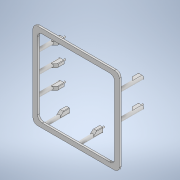
# Autodesk Inventor part: Jig
Saved by Autodesk Inventor 2022.3 (Build 263350030, 350C)
## iProperties
Created: 2023-05-04
Part Number: Jig
Material: Generic
Document SubType Name: Modeling
Designer: Ben
Density: 1 g/cm^3
Appearance: Default
Author: Ben
Autodesk Inventor part; units mm, degrees
(part 1 of 2)
ref_plane "Work Plane1" through (0, 0, 25) normal (0, 0, 1) x (1, 0, 0)
sketch "Sketch1" plane through (0, 0, 25) normal (0, 0, 1) x (1, 0, 0)
  line L0 (46.5, -46.5) -> (-46.5, -46.5)
  line L1 (-46.5, -46.5) -> (-46.5, 46.5)
  line L2 (-46.5, 46.5) -> (46.5, 46.5)
  line L3 (46.5, 46.5) -> (46.5, -46.5)
  line L4 (46.5, -46.5) -> (-46.5, 46.5) construction
  line L5 (-46.5, -46.5) -> (46.5, 46.5) construction
  line L6 (-41.5, 41.5) -> (41.5, 41.5)
  line L7 (41.5, 41.5) -> (41.5, -41.5)
  line L8 (41.5, -41.5) -> (-41.5, -41.5)
  line L9 (-41.5, -41.5) -> (-41.5, 41.5)
  line L10 (-41.5, 41.5) -> (41.5, -41.5) construction
  line L11 (41.5, 41.5) -> (-41.5, -41.5) construction
  point P0 (0, 0)
  dimension "d0" = 93
  dimension "d1" = 93
  dimension "d2" = 83
  dimension "d3" = 83
  constraints: 24 end point, 4 midpoint, 4 parallel, 2 horizontal, 2 perpendicular
  measures "d0" distance of L1.end L2.end
  measures "d1" distance of L0.end L1.end
  measures "d2" distance of L7.end L8.end
  measures "d3" distance of L6.end L7.end
extrude "Extrusion1" add sketch "Sketch1" along normal blind 2
sketch "Sketch2" plane through (0, 0, 25) normal (0, 0, -1) x (-1, 0, 0)
  line L0 (42.0226, -36.7562) -> (42.0242, -37.0987) projected
  line L1 (42.0242, -37.0987) -> (41.9381, -37.7782) projected
  line L2 (41.9381, -37.7782) -> (41.764, -38.4406) projected
  line L3 (41.764, -38.4406) -> (41.5049, -39.0746) projected
  line L4 (41.5049, -39.0746) -> (41.1653, -39.6694) projected
  line L5 (41.1653, -39.6694) -> (40.7509, -40.2148) projected
  line L6 (40.7509, -40.2148) -> (40.2689, -40.7015) projected
  line L7 (40.2689, -40.7015) -> (39.7275, -41.121) projected
  line L8 (39.7275, -41.121) -> (39.136, -41.4663) projected
  line L9 (39.136, -41.4663) -> (38.5044, -41.7315) projected
  line L10 (38.5044, -41.7315) -> (37.8437, -41.9119) projected
  line L11 (37.8437, -41.9119) -> (37.165, -42.0046) projected
  line L12 (37.165, -42.0046) -> (36.8226, -42.0062) projected
  line L13 (36.8226, -42.0062) -> (36.7976, -42.0062) projected
  line L14 (36.7976, -42.0062) -> (22.0476, -42.0062) projected
  line L15 (22.0476, -42.0062) -> (22.039, -41.8757) projected
  line L16 (22.039, -41.8757) -> (21.9715, -41.6235) projected
  line L17 (21.9715, -41.6235) -> (21.8409, -41.3974) projected
  line L18 (21.8409, -41.3974) -> (21.6563, -41.2129) projected
  line L19 (21.6563, -41.2129) -> (21.4303, -41.0823) projected
  line L20 (21.4303, -41.0823) -> (21.1781, -41.0148) projected
  line L21 (21.1781, -41.0148) -> (20.9171, -41.0148) projected
  line L22 (20.9171, -41.0148) -> (20.6649, -41.0823) projected
  line L23 (20.6649, -41.0823) -> (20.4388, -41.2129) projected
  line L24 (20.4388, -41.2129) -> (20.2543, -41.3974) projected
  line L25 (20.2543, -41.3974) -> (20.1237, -41.6235) projected
  line L26 (20.1237, -41.6235) -> (20.0562, -41.8757) projected
  line L27 (20.0562, -41.8757) -> (20.0476, -42.0062) projected
  line L28 (20.0476, -42.0062) -> (1.0226, -42.0062) projected
  line L29 (1.0226, -42.0062) -> (1.014, -41.8757) projected
  line L30 (1.014, -41.8757) -> (0.9465, -41.6235) projected
  line L31 (0.9465, -41.6235) -> (0.8159, -41.3974) projected
  line L32 (0.8159, -41.3974) -> (0.6313, -41.2129) projected
  line L33 (0.6313, -41.2129) -> (0.4053, -41.0823) projected
  line L34 (0.4053, -41.0823) -> (0.1531, -41.0148) projected
  line L35 (0.1531, -41.0148) -> (-0.1079, -41.0148) projected
  line L36 (-0.1079, -41.0148) -> (-0.3601, -41.0823) projected
  line L37 (-0.3601, -41.0823) -> (-0.5862, -41.2129) projected
  line L38 (-0.5862, -41.2129) -> (-0.7707, -41.3974) projected
  line L39 (-0.7707, -41.3974) -> (-0.9013, -41.6235) projected
  line L40 (-0.9013, -41.6235) -> (-0.9688, -41.8757) projected
  line L41 (-0.9688, -41.8757) -> (-0.9774, -42.0062) projected
  line L42 (-0.9774, -42.0062) -> (-19.9774, -42.0062) projected
  line L43 (-19.9774, -42.0062) -> (-19.986, -41.8757) projected
  line L44 (-19.986, -41.8757) -> (-20.0536, -41.6235) projected
  line L45 (-20.0536, -41.6235) -> (-20.1841, -41.3975) projected
  line L46 (-20.1841, -41.3975) -> (-20.3687, -41.2129) projected
  line L47 (-20.3687, -41.2129) -> (-20.5947, -41.0823) projected
  line L48 (-20.5947, -41.0823) -> (-20.8469, -41.0148) projected
  line L49 (-20.8469, -41.0148) -> (-21.1079, -41.0148) projected
  line L50 (-21.1079, -41.0148) -> (-21.3601, -41.0823) projected
  line L51 (-21.3601, -41.0823) -> (-21.5862, -41.2129) projected
  line L52 (-21.5862, -41.2129) -> (-21.7707, -41.3975) projected
  line L53 (-21.7707, -41.3975) -> (-21.9013, -41.6235) projected
  line L54 (-21.9013, -41.6235) -> (-21.9688, -41.8757) projected
  line L55 (-21.9688, -41.8757) -> (-21.9774, -42.0062) projected
  line L56 (-21.9774, -42.0062) -> (-36.7274, -42.0062) projected
  line L57 (-36.7274, -42.0062) -> (-37.0699, -42.0079) projected
  line L58 (-37.0699, -42.0079) -> (-37.7494, -41.9217) projected
  line L59 (-37.7494, -41.9217) -> (-38.4118, -41.7476) projected
  line L60 (-38.4118, -41.7476) -> (-39.0459, -41.4885) projected
  line L61 (-39.0459, -41.4885) -> (-39.6407, -41.1489) projected
  line L62 (-39.6407, -41.1489) -> (-40.186, -40.7345) projected
  line L63 (-40.186, -40.7345) -> (-40.6727, -40.2525) projected
  line L64 (-40.6727, -40.2525) -> (-41.0922, -39.7111) projected
  line L65 (-41.0922, -39.7111) -> (-41.4375, -39.1196) projected
  line L66 (-41.4375, -39.1196) -> (-41.7027, -38.4881) projected
  line L67 (-41.7027, -38.4881) -> (-41.8831, -37.8273) projected
  line L68 (-41.8831, -37.8273) -> (-41.9758, -37.1487) projected
  line L69 (-41.9758, -37.1487) -> (-41.9774, -36.8062) projected
  line L70 (-41.9774, -36.8062) -> (-41.9524, -36.7812) projected
  line L71 (-41.9524, -36.7812) -> (-41.9524, -22.0312) projected
  line L72 (-41.9524, -22.0312) -> (-41.8219, -22.0226) projected
  line L73 (-41.8219, -22.0226) -> (-41.5697, -21.9551) projected
  line L74 (-41.5697, -21.9551) -> (-41.3437, -21.8246) projected
  line L75 (-41.3437, -21.8246) -> (-41.1591, -21.64) projected
  line L76 (-41.1591, -21.64) -> (-41.0285, -21.4139) projected
  line L77 (-41.0285, -21.4139) -> (-40.961, -21.1617) projected
  line L78 (-40.961, -21.1617) -> (-40.961, -20.9007) projected
  line L79 (-40.961, -20.9007) -> (-41.0285, -20.6485) projected
  line L80 (-41.0285, -20.6485) -> (-41.1591, -20.4225) projected
  line L81 (-41.1591, -20.4225) -> (-41.3436, -20.2379) projected
  line L82 (-41.3436, -20.2379) -> (-41.5697, -20.1073) projected
  line L83 (-41.5697, -20.1073) -> (-41.8219, -20.0398) projected
  line L84 (-41.8219, -20.0398) -> (-41.9524, -20.0312) projected
  line L85 (-41.9524, -20.0312) -> (-41.9524, -1.0062) projected
  line L86 (-41.9524, -1.0062) -> (-41.8219, -0.9976) projected
  line L87 (-41.8219, -0.9976) -> (-41.5697, -0.9301) projected
  line L88 (-41.5697, -0.9301) -> (-41.3437, -0.7996) projected
  line L89 (-41.3437, -0.7996) -> (-41.1591, -0.615) projected
  line L90 (-41.1591, -0.615) -> (-41.0285, -0.3889) projected
  line L91 (-41.0285, -0.3889) -> (-40.961, -0.1367) projected
  line L92 (-40.961, -0.1367) -> (-40.961, 0.1243) projected
  line L93 (-40.961, 0.1243) -> (-41.0285, 0.3765) projected
  line L94 (-41.0285, 0.3765) -> (-41.1591, 0.6025) projected
  line L95 (-41.1591, 0.6025) -> (-41.3436, 0.7871) projected
  line L96 (-41.3436, 0.7871) -> (-41.5697, 0.9177) projected
  line L97 (-41.5697, 0.9177) -> (-41.8219, 0.9852) projected
  line L98 (-41.8219, 0.9852) -> (-41.9524, 0.9938) projected
  line L99 (-41.9524, 0.9938) -> (-41.9524, 19.9938) projected
  line L100 (-41.9524, 19.9938) -> (-41.8219, 20.0024) projected
  line L101 (-41.8219, 20.0024) -> (-41.5697, 20.0699) projected
  line L102 (-41.5697, 20.0699) -> (-41.3437, 20.2005) projected
  line L103 (-41.3437, 20.2005) -> (-41.1591, 20.385) projected
  line L104 (-41.1591, 20.385) -> (-41.0286, 20.6111) projected
  line L105 (-41.0286, 20.6111) -> (-40.961, 20.8633) projected
  line L106 (-40.961, 20.8633) -> (-40.961, 21.1243) projected
  line L107 (-40.961, 21.1243) -> (-41.0285, 21.3765) projected
  line L108 (-41.0285, 21.3765) -> (-41.1591, 21.6025) projected
  line L109 (-41.1591, 21.6025) -> (-41.3437, 21.7871) projected
  line L110 (-41.3437, 21.7871) -> (-41.5697, 21.9177) projected
  line L111 (-41.5697, 21.9177) -> (-41.8219, 21.9852) projected
  line L112 (-41.8219, 21.9852) -> (-41.9524, 21.9938) projected
  line L113 (-41.9524, 21.9938) -> (-41.9524, 36.7438) projected
  line L114 (-41.9524, 36.7438) -> (-41.9541, 37.0862) projected
  line L115 (-41.9541, 37.0862) -> (-41.8679, 37.7657) projected
  line L116 (-41.8679, 37.7657) -> (-41.6938, 38.4282) projected
  line L117 (-41.6938, 38.4282) -> (-41.4347, 39.0622) projected
  line L118 (-41.4347, 39.0622) -> (-41.0951, 39.657) projected
  line L119 (-41.0951, 39.657) -> (-40.6807, 40.2024) projected
  line L120 (-40.6807, 40.2024) -> (-40.1987, 40.6891) projected
  line L121 (-40.1987, 40.6891) -> (-39.6573, 41.1086) projected
  line L122 (-39.6573, 41.1086) -> (-39.0658, 41.4539) projected
  line L123 (-39.0658, 41.4539) -> (-38.4343, 41.7191) projected
  line L124 (-38.4343, 41.7191) -> (-37.7735, 41.8995) projected
  line L125 (-37.7735, 41.8995) -> (-37.0949, 41.9922) projected
  line L126 (-37.0949, 41.9922) -> (-36.7524, 41.9938) projected
  line L127 (-36.7524, 41.9938) -> (-22.0024, 41.9938) projected
  line L128 (-22.0024, 41.9938) -> (-21.9939, 41.8633) projected
  line L129 (-21.9939, 41.8633) -> (-21.9263, 41.6111) projected
  line L130 (-21.9263, 41.6111) -> (-21.7958, 41.385) projected
  line L131 (-21.7958, 41.385) -> (-21.6112, 41.2004) projected
  line L132 (-21.6112, 41.2004) -> (-21.3851, 41.0699) projected
  line L133 (-21.3851, 41.0699) -> (-21.1329, 41.0024) projected
  line L134 (-21.1329, 41.0024) -> (-20.8719, 41.0024) projected
  line L135 (-20.8719, 41.0024) -> (-20.6197, 41.0699) projected
  line L136 (-20.6197, 41.0699) -> (-20.3937, 41.2004) projected
  line L137 (-20.3937, 41.2004) -> (-20.2091, 41.385) projected
  line L138 (-20.2091, 41.385) -> (-20.0785, 41.6111) projected
  line L139 (-20.0785, 41.6111) -> (-20.011, 41.8633) projected
  line L140 (-20.011, 41.8633) -> (-20.0024, 41.9938) projected
  line L141 (-20.0024, 41.9938) -> (-0.9774, 41.9938) projected
  line L142 (-0.9774, 41.9938) -> (-0.9689, 41.8633) projected
  line L143 (-0.9689, 41.8633) -> (-0.9013, 41.6111) projected
  line L144 (-0.9013, 41.6111) -> (-0.7708, 41.385) projected
  line L145 (-0.7708, 41.385) -> (-0.5862, 41.2004) projected
  line L146 (-0.5862, 41.2004) -> (-0.3601, 41.0699) projected
  line L147 (-0.3601, 41.0699) -> (-0.1079, 41.0024) projected
  line L148 (-0.1079, 41.0024) -> (0.1531, 41.0024) projected
  line L149 (0.1531, 41.0024) -> (0.4053, 41.0699) projected
  line L150 (0.4053, 41.0699) -> (0.6313, 41.2005) projected
  line L151 (0.6313, 41.2005) -> (0.8159, 41.385) projected
  line L152 (0.8159, 41.385) -> (0.9465, 41.6111) projected
  line L153 (0.9465, 41.6111) -> (1.014, 41.8633) projected
  line L154 (1.014, 41.8633) -> (1.0226, 41.9938) projected
  line L155 (1.0226, 41.9938) -> (20.0226, 41.9938) projected
  line L156 (20.0226, 41.9938) -> (20.0312, 41.8633) projected
  line L157 (20.0312, 41.8633) -> (20.0987, 41.6111) projected
  line L158 (20.0987, 41.6111) -> (20.2292, 41.385) projected
  line L159 (20.2292, 41.385) -> (20.4138, 41.2005) projected
  line L160 (20.4138, 41.2005) -> (20.6399, 41.0699) projected
  line L161 (20.6399, 41.0699) -> (20.8921, 41.0024) projected
  line L162 (20.8921, 41.0024) -> (21.1531, 41.0024) projected
  line L163 (21.1531, 41.0024) -> (21.4053, 41.0699) projected
  line L164 (21.4053, 41.0699) -> (21.6313, 41.2005) projected
  line L165 (21.6313, 41.2005) -> (21.8159, 41.385) projected
  line L166 (21.8159, 41.385) -> (21.9465, 41.6111) projected
  line L167 (21.9465, 41.6111) -> (22.014, 41.8633) projected
  line L168 (22.014, 41.8633) -> (22.0226, 41.9938) projected
  line L169 (22.0226, 41.9938) -> (36.7726, 41.9938) projected
  line L170 (36.7726, 41.9938) -> (37.115, 41.9955) projected
  line L171 (37.115, 41.9955) -> (37.7945, 41.9093) projected
  line L172 (37.7945, 41.9093) -> (38.457, 41.7352) projected
  line L173 (38.457, 41.7352) -> (39.091, 41.4761) projected
  line L174 (39.091, 41.4761) -> (39.6858, 41.1365) projected
  line L175 (39.6858, 41.1365) -> (40.2312, 40.7221) projected
  line L176 (40.2312, 40.7221) -> (40.7179, 40.2401) projected
  line L177 (40.7179, 40.2401) -> (41.1374, 39.6987) projected
  line L178 (41.1374, 39.6987) -> (41.4827, 39.1072) projected
  line L179 (41.4827, 39.1072) -> (41.7479, 38.4756) projected
  line L180 (41.7479, 38.4756) -> (41.9283, 37.8149) projected
  line L181 (41.9283, 37.8149) -> (42.0209, 37.1363) projected
  line L182 (42.0209, 37.1363) -> (42.0226, 36.7938) projected
  line L183 (42.0226, 36.7938) -> (42.0226, 36.7688) projected
  line L184 (42.0226, 36.7688) -> (42.0226, 22.0188) projected
  line L185 (42.0226, 22.0188) -> (41.8921, 22.0102) projected
  line L186 (41.8921, 22.0102) -> (41.6399, 21.9427) projected
  line L187 (41.6399, 21.9427) -> (41.4138, 21.8121) projected
  line L188 (41.4138, 21.8121) -> (41.2292, 21.6276) projected
  line L189 (41.2292, 21.6276) -> (41.0987, 21.4015) projected
  line L190 (41.0987, 21.4015) -> (41.0312, 21.1493) projected
  line L191 (41.0312, 21.1493) -> (41.0312, 20.8883) projected
  line L192 (41.0312, 20.8883) -> (41.0987, 20.6361) projected
  line L193 (41.0987, 20.6361) -> (41.2292, 20.41) projected
  line L194 (41.2292, 20.41) -> (41.4138, 20.2255) projected
  line L195 (41.4138, 20.2255) -> (41.6399, 20.0949) projected
  line L196 (41.6399, 20.0949) -> (41.8921, 20.0274) projected
  line L197 (41.8921, 20.0274) -> (42.0226, 20.0188) projected
  line L198 (42.0226, 20.0188) -> (42.0226, 0.9938) projected
  line L199 (42.0226, 0.9938) -> (41.8921, 0.9852) projected
  line L200 (41.8921, 0.9852) -> (41.6399, 0.9177) projected
  line L201 (41.6399, 0.9177) -> (41.4138, 0.7871) projected
  line L202 (41.4138, 0.7871) -> (41.2292, 0.6026) projected
  line L203 (41.2292, 0.6026) -> (41.0987, 0.3765) projected
  line L204 (41.0987, 0.3765) -> (41.0312, 0.1243) projected
  line L205 (41.0312, 0.1243) -> (41.0312, -0.1367) projected
  line L206 (41.0312, -0.1367) -> (41.0987, -0.3889) projected
  line L207 (41.0987, -0.3889) -> (41.2293, -0.615) projected
  line L208 (41.2293, -0.615) -> (41.4138, -0.7995) projected
  line L209 (41.4138, -0.7995) -> (41.6399, -0.9301) projected
  line L210 (41.6399, -0.9301) -> (41.8921, -0.9976) projected
  line L211 (41.8921, -0.9976) -> (42.0226, -1.0062) projected
  line L212 (42.0226, -1.0062) -> (42.0226, -20.0062) projected
  line L213 (42.0226, -20.0062) -> (41.8921, -20.0148) projected
  line L214 (41.8921, -20.0148) -> (41.6399, -20.0823) projected
  line L215 (41.6399, -20.0823) -> (41.4138, -20.2129) projected
  line L216 (41.4138, -20.2129) -> (41.2293, -20.3975) projected
  line L217 (41.2293, -20.3975) -> (41.0987, -20.6235) projected
  line L218 (41.0987, -20.6235) -> (41.0312, -20.8757) projected
  line L219 (41.0312, -20.8757) -> (41.0312, -21.1367) projected
  line L220 (41.0312, -21.1367) -> (41.0987, -21.3889) projected
  line L221 (41.0987, -21.3889) -> (41.2293, -21.615) projected
  line L222 (41.2293, -21.615) -> (41.4139, -21.7995) projected
  line L223 (41.4139, -21.7995) -> (41.6399, -21.9301) projected
  line L224 (41.6399, -21.9301) -> (41.8921, -21.9976) projected
  line L225 (41.8921, -21.9976) -> (42.0226, -22.0062) projected
  line L226 (42.0226, -22.0062) -> (42.0226, -36.7562) projected
  circle A0 centre (-20.9774, -0.0062) radius 1.2055 projected
  circle A1 centre (0.0226, 20.9938) radius 1.2055 projected
  circle A2 centre (0.0226, -21.0062) radius 1.2055 projected
  circle A3 centre (0.0226, -0.0062) radius 1.2055 projected
  circle A4 centre (21.0226, -0.0062) radius 1.2055 projected
  circle A5 centre (36.7726, -34.2562) radius 0.4555 projected
  circle A6 centre (36.7726, -39.2562) radius 0.4555 projected
  circle A7 centre (26.2726, -34.2562) radius 0.4555 projected
  circle A8 centre (26.2726, -39.2562) radius 0.4555 projected
  circle A9 centre (-15.7274, 28.7438) radius 0.4555 projected
  circle A10 centre (-15.7274, 23.7438) radius 0.4555 projected
  circle A11 centre (-36.7274, 23.7438) radius 0.4555 projected
  circle A12 centre (-36.7274, 28.7438) radius 0.4555 projected
  circle A13 centre (26.2726, 39.2438) radius 0.4555 projected
  circle A14 centre (26.2726, 34.2438) radius 0.4555 projected
  circle A15 centre (5.2726, 34.2438) radius 0.4555 projected
  circle A16 centre (5.2726, 39.2438) radius 0.4555 projected
  circle A17 centre (-15.7274, 39.2438) radius 0.4555 projected
  circle A18 centre (-15.7274, 34.2438) radius 0.4555 projected
  circle A19 centre (-36.7274, 34.2438) radius 0.4555 projected
  circle A20 centre (-36.7274, 39.2438) radius 0.4555 projected
  circle A21 centre (5.2726, -34.2562) radius 0.4555 projected
  circle A22 centre (5.2726, -39.2562) radius 0.4555 projected
  circle A23 centre (-15.7274, -39.2562) radius 0.4555 projected
  circle A24 centre (-15.7274, -34.2562) radius 0.4555 projected
  circle A25 centre (-36.7274, -34.2562) radius 0.4555 projected
  circle A26 centre (-36.7274, -39.2562) radius 0.4555 projected
  circle A27 centre (26.2726, -28.7562) radius 0.4555 projected
  circle A28 centre (26.2726, -23.7562) radius 0.4555 projected
  circle A29 centre (5.2726, -23.7562) radius 0.4555 projected
  circle A30 centre (5.2726, -28.7562) radius 0.4555 projected
  circle A31 centre (-15.7274, -28.7562) radius 0.4555 projected
  circle A32 centre (-15.7274, -23.7562) radius 0.4555 projected
  circle A33 centre (-36.7274, -23.7562) radius 0.4555 projected
  circle A34 centre (-36.7274, -28.7562) radius 0.4555 projected
  circle A35 centre (26.2726, -18.2562) radius 0.4555 projected
  circle A36 centre (26.2726, -13.2562) radius 0.4555 projected
  circle A37 centre (5.2726, -13.2562) radius 0.4555 projected
  circle A38 centre (5.2726, -18.2562) radius 0.4555 projected
  circle A39 centre (-15.7274, -18.2562) radius 0.4555 projected
  circle A40 centre (-15.7274, -13.2562) radius 0.4555 projected
  circle A41 centre (-36.7274, -13.2562) radius 0.4555 projected
  circle A42 centre (-36.7274, -18.2562) radius 0.4555 projected
  circle A43 centre (26.2726, -7.7562) radius 0.4555 projected
  circle A44 centre (26.2726, -2.7562) radius 0.4555 projected
  circle A45 centre (5.2726, -2.7562) radius 0.4555 projected
  circle A46 centre (5.2726, -7.7562) radius 0.4555 projected
  circle A47 centre (-15.7274, -7.7562) radius 0.4555 projected
  circle A48 centre (-15.7274, -2.7562) radius 0.4555 projected
  circle A49 centre (-36.7274, -2.7562) radius 0.4555 projected
  circle A50 centre (-36.7274, -7.7562) radius 0.4555 projected
  circle A51 centre (26.2726, 2.7438) radius 0.4555 projected
  circle A52 centre (26.2726, 7.7438) radius 0.4555 projected
  circle A53 centre (5.2726, 7.7438) radius 0.4555 projected
  circle A54 centre (5.2726, 2.7438) radius 0.4555 projected
  circle A55 centre (-15.7274, 2.7438) radius 0.4555 projected
  circle A56 centre (-15.7274, 7.7438) radius 0.4555 projected
  circle A57 centre (-36.7274, 7.7438) radius 0.4555 projected
  circle A58 centre (-36.7274, 2.7438) radius 0.4555 projected
  circle A59 centre (26.2726, 13.2438) radius 0.4555 projected
  circle A60 centre (26.2726, 18.2438) radius 0.4555 projected
  circle A61 centre (5.2726, 18.2438) radius 0.4555 projected
  circle A62 centre (5.2726, 13.2438) radius 0.4555 projected
  circle A63 centre (-15.7274, 13.2438) radius 0.4555 projected
  circle A64 centre (-15.7274, 18.2438) radius 0.4555 projected
  circle A65 centre (-36.7274, 18.2438) radius 0.4555 projected
  circle A66 centre (-36.7274, 13.2438) radius 0.4555 projected
  circle A67 centre (26.2726, 23.7438) radius 0.4555 projected
  circle A68 centre (26.2726, 28.7438) radius 0.4555 projected
  circle A69 centre (5.2726, 28.7438) radius 0.4555 projected
  circle A70 centre (5.2726, 23.7438) radius 0.4555 projected
  circle A71 centre (-5.2274, 23.7438) radius 0.4555 projected
  circle A72 centre (-5.2274, 28.7438) radius 0.4555 projected
  circle A73 centre (-26.2274, 28.7438) radius 0.4555 projected
  circle A74 centre (-26.2274, 23.7438) radius 0.4555 projected
  circle A75 centre (36.7726, 34.2438) radius 0.4555 projected
  circle A76 centre (36.7726, 39.2438) radius 0.4555 projected
  circle A77 centre (15.7726, 39.2438) radius 0.4555 projected
  circle A78 centre (15.7726, 34.2438) radius 0.4555 projected
  circle A79 centre (-5.2274, 34.2438) radius 0.4555 projected
  circle A80 centre (-5.2274, 39.2438) radius 0.4555 projected
  circle A81 centre (-26.2274, 39.2438) radius 0.4555 projected
  circle A82 centre (-26.2274, 34.2438) radius 0.4555 projected
  circle A83 centre (15.7726, -39.2562) radius 0.4555 projected
  circle A84 centre (15.7726, -34.2562) radius 0.4555 projected
  circle A85 centre (-5.2274, -34.2562) radius 0.4555 projected
  circle A86 centre (-5.2274, -39.2562) radius 0.4555 projected
  circle A87 centre (-26.2274, -39.2562) radius 0.4555 projected
  circle A88 centre (-26.2274, -34.2562) radius 0.4555 projected
  circle A89 centre (36.7726, -23.7562) radius 0.4555 projected
  circle A90 centre (36.7726, -28.7562) radius 0.4555 projected
  circle A91 centre (15.7726, -28.7562) radius 0.4555 projected
  circle A92 centre (15.7726, -23.7562) radius 0.4555 projected
  circle A93 centre (-5.2274, -23.7562) radius 0.4555 projected
  circle A94 centre (-5.2274, -28.7562) radius 0.4555 projected
  circle A95 centre (-26.2274, -28.7562) radius 0.4555 projected
  circle A96 centre (-26.2274, -23.7562) radius 0.4555 projected
  circle A97 centre (36.7726, -13.2562) radius 0.4555 projected
  circle A98 centre (36.7726, -18.2562) radius 0.4555 projected
  circle A99 centre (15.7726, -18.2562) radius 0.4555 projected
  circle A100 centre (15.7726, -13.2562) radius 0.4555 projected
  circle A101 centre (-5.2274, -13.2562) radius 0.4555 projected
  circle A102 centre (-5.2274, -18.2562) radius 0.4555 projected
  circle A103 centre (-26.2274, -18.2562) radius 0.4555 projected
  circle A104 centre (-26.2274, -13.2562) radius 0.4555 projected
  circle A105 centre (36.7726, -2.7562) radius 0.4555 projected
  circle A106 centre (36.7726, -7.7562) radius 0.4555 projected
  circle A107 centre (15.7726, -7.7562) radius 0.4555 projected
  circle A108 centre (15.7726, -2.7562) radius 0.4555 projected
  circle A109 centre (-5.2274, -2.7562) radius 0.4555 projected
  circle A110 centre (-5.2274, -7.7562) radius 0.4555 projected
  circle A111 centre (-26.2274, -7.7562) radius 0.4555 projected
  circle A112 centre (-26.2274, -2.7562) radius 0.4555 projected
  circle A113 centre (36.7726, 7.7438) radius 0.4555 projected
  circle A114 centre (36.7726, 2.7438) radius 0.4555 projected
  circle A115 centre (15.7726, 2.7438) radius 0.4555 projected
  circle A116 centre (15.7726, 7.7438) radius 0.4555 projected
  circle A117 centre (-5.2274, 7.7438) radius 0.4555 projected
  circle A118 centre (-5.2274, 2.7438) radius 0.4555 projected
  circle A119 centre (-26.2274, 2.7438) radius 0.4555 projected
  circle A120 centre (-26.2274, 7.7438) radius 0.4555 projected
  circle A121 centre (36.7726, 18.2438) radius 0.4555 projected
  circle A122 centre (36.7726, 13.2438) radius 0.4555 projected
  circle A123 centre (15.7726, 13.2438) radius 0.4555 projected
  circle A124 centre (15.7726, 18.2438) radius 0.4555 projected
  circle A125 centre (-5.2274, 18.2438) radius 0.4555 projected
  circle A126 centre (-5.2274, 13.2438) radius 0.4555 projected
  circle A127 centre (-26.2274, 13.2438) radius 0.4555 projected
  circle A128 centre (-26.2274, 18.2438) radius 0.4555 projected
  circle A129 centre (36.7726, 28.7438) radius 0.4555 projected
  circle A130 centre (36.7726, 23.7438) radius 0.4555 projected
  circle A131 centre (15.7726, 23.7438) radius 0.4555 projected
  circle A132 centre (15.7726, 28.7438) radius 0.4555 projected
  circle A133 centre (-44.061, -28.0062) radius 1.9
  circle A134 centre (-44.061, -0.0062) radius 1.9
  circle A135 centre (-44.061, 27.9938) radius 1.9
  circle A136 centre (36.0226, -44.1104) radius 1.9
  circle A137 centre (0.0226, -44.1104) radius 1.9
  circle A138 centre (-14.9774, -44.3108) radius 1.9
  circle A139 centre (44.1391, -21.0282) radius 1.9
  circle A140 centre (44.1391, -0.0282) radius 1.9
  circle A141 centre (43.9387, 21.1023) radius 1.9
  circle A142 centre (21.0564, 44.1024) radius 1.9
  circle A143 centre (0.0226, 44.1026) radius 1.9
  circle A144 centre (-21.0741, 43.902) radius 1.9
  line L227 (0.0226, 41.0024) -> (0.0226, 44.1026) construction
  line L228 (-44.061, -0.0062) -> (-40.961, -0.0062) construction
  point P0 (0, 0)
  dimension "d6" = 3.8
  dimension "d7" = 3.8
  dimension "d8" = 3.8
  dimension "d9" = 3.8
  dimension "d10" = 3.8
  dimension "d11" = 3.8
  dimension "d12" = 3.8
  dimension "d13" = 3.8
  dimension "d14" = 3.8
  dimension "d15" = 3.8
  dimension "d16" = 3.8
  dimension "d17" = 3.8
  dimension "d18" = 3.1
  dimension "d21" = 28
  dimension "d22" = 28
  dimension "d23" = 15
  dimension "d24" = 36
  constraints: 12 centre point, 4 end point, 2 midpoint, 2 vertical alignment, 1 vertical
  measures "d6" diameter of A133
  measures "d7" diameter of A134
  measures "d8" diameter of A135
  measures "d9" diameter of A136
  measures "d10" diameter of A137
  measures "d11" diameter of A138
  measures "d12" diameter of A139
  measures "d13" diameter of A140
  measures "d14" diameter of A141
  measures "d15" diameter of A142
  measures "d16" diameter of A143
  measures "d17" diameter of A144
  measures "d18" distance of L228.start L228.end
  measures "d21" distance of A133.centre L228.start
  measures "d22" distance of L228.start A135.centre
  measures "d23" horizontal distance of A138.centre A137.centre
  measures "d24" distance of A136.centre A137.centre
ref_plane "Work Plane2" through (-42.0243, -42.0079, -11.537) normal (0, 0, 1) x (1, 0, 0)
ref_plane "Work Plane3" through (-42.0017, -42.0001, 0) normal (0, 0, 1) x (1, 0, 0)
extrude "Extrusion2" add sketch "Sketch2" along normal up to surface (25 mm away) contours A134 | A135 | A136 | A137 | A139 | A140 | A141
sketch "Sketch3" plane through (-0.0226, -44.1104, 0) normal (0, 0, -1) x (-1, 0, 0)
  circle A0 centre (43.9161, 65.2127) radius 1.9 projected
  line L0 (43.9161, 63.3127) -> (43.9161, 67.1127)
  line L1 (43.9161, 67.1127) -> (39.6386, 67.1127)
  line L2 (39.6386, 67.1127) -> (39.6386, 63.3127)
  line L3 (39.6386, 63.3127) -> (43.9161, 63.3127)
  circle A1 centre (43.9161, 65.2127) radius 1.9 projected
  circle A2 centre (44.1165, 44.0822) radius 1.9 projected
  circle A3 centre (44.1165, 23.0822) radius 1.9 projected
  circle A4 centre (-44.0836, 72.1042) radius 1.9 projected
  circle A5 centre (-44.0836, 44.1042) radius 1.9 projected
  circle A6 centre (0, 0) radius 1.9 projected
  circle A7 centre (36, 0) radius 1.9 projected
  line L4 (44.1165, 42.1822) -> (44.1165, 45.9822)
  line L5 (44.1165, 45.9822) -> (39.839, 45.9822)
  line L6 (39.839, 45.9822) -> (39.839, 42.1822)
  line L7 (39.839, 42.1822) -> (44.1165, 42.1822)
  line L8 (43.9161, 21.1822) -> (43.9161, 24.9822)
  line L9 (43.9161, 24.9822) -> (39.6386, 24.9822)
  line L10 (39.6386, 24.9822) -> (39.6386, 21.1822)
  line L11 (39.6386, 21.1822) -> (43.9161, 21.1822)
  line L12 (-39.8251, 45.9936) -> (-44.1026, 45.9936)
  line L13 (-44.1026, 45.9936) -> (-44.1026, 42.1936)
  line L14 (-44.1026, 42.1936) -> (-39.8251, 42.1936)
  line L15 (-39.8251, 42.1936) -> (-39.8251, 45.9936)
  line L16 (-39.8583, 74.0042) -> (-44.1358, 74.0042)
  line L17 (-44.1358, 74.0042) -> (-44.1358, 70.223)
  line L18 (-44.1358, 70.223) -> (-39.8583, 70.223)
  line L19 (-39.8583, 70.223) -> (-39.8583, 74.0042)
  circle A8 centre (36, 0) radius 1.9 projected
  line L20 (37.9, 0) -> (34.1, 0)
  line L21 (34.1, 0) -> (34.1, 4.3653)
  line L22 (34.1, 4.3653) -> (37.9, 4.3653)
  line L23 (37.9, 4.3653) -> (37.9, 0)
  circle A9 centre (0, 0) radius 1.9 projected
  line L24 (1.9, 0) -> (1.9, 4.3653)
  line L25 (1.9, 4.3653) -> (-1.9, 4.3653)
  line L26 (-1.9, 4.3653) -> (-1.9, 0)
  point P0 (-0.0226, 44.1104)
  point P1 (-43.8832, 45.9936)
  point P2 (-44.1026, 42.2043)
  point P3 (-44.0836, 74.0042)
  point P4 (-43.8169, 70.223)
  point P5 (43.9161, 21.1928)
  point P6 (43.9161, 24.9716)
  point P7 (1.9, 0)
  constraints: 54 end point, 12 perpendicular, 6 horizontal, 6 point on circle, 6 tangent, 6 vertical, 4 point on line, 1 parallel
extrude "Extrusion3" add sketch "Sketch3" against normal blind 10 contours A0 L3 L2 L1 | A2 L7 L6 L5 | A3 L8 L11 L10 L9 | A4 L16 L19 L18 | A5 L12 L15 L14 L13 | A6 L26 L25 L24 | A7 L21 L22 L23
sketch "Sketch4" plane through (44.061, 29.8938, 0) normal (0, 0, -1) x (-1, 0, 0)
  arc A0 (0.2004, -28.0106) -> (-0.019, -31.7999) centre (0, -29.9) ccw projected
  line L0 (-0.019, -31.7999) -> (-0.019, -31.8106) projected
  line L1 (-0.019, -31.8106) -> (4.2585, -31.8106) projected
  line L2 (4.2585, -31.8106) -> (4.2585, -28.0106) projected
  line L3 (4.2585, -28.0106) -> (0.2004, -28.0106) projected
  arc A1 (0, 0) -> (0.2667, -3.7812) centre (0, -1.9) ccw projected
  line L4 (0.2667, -3.7812) -> (4.2252, -3.7812) projected
  line L5 (4.2252, -3.7812) -> (4.2252, 0) projected
  line L6 (4.2252, 0) -> (0, 0) projected
  arc A2 (87.9997, -10.6915) -> (87.9997, -6.8915) centre (87.9997, -8.7915) ccw projected
  line L7 (87.9997, -6.8915) -> (83.7222, -6.8915) projected
  line L8 (83.7222, -6.8915) -> (83.7222, -10.6915) projected
  line L9 (83.7222, -10.6915) -> (87.9997, -10.6915) projected
  arc A3 (88.2001, -31.822) -> (88.2001, -28.022) centre (88.2001, -29.922) ccw projected
  line L10 (88.2001, -28.022) -> (83.9226, -28.022) projected
  line L11 (83.9226, -28.022) -> (83.9226, -31.822) projected
  line L12 (83.9226, -31.822) -> (88.2001, -31.822) projected
  arc A4 (87.9997, -52.8114) -> (87.9997, -49.0326) centre (88.2001, -50.922) ccw projected
  line L13 (87.9997, -49.0326) -> (87.9997, -49.022) projected
  line L14 (87.9997, -49.022) -> (83.7222, -49.022) projected
  line L15 (83.7222, -49.022) -> (83.7222, -52.822) projected
  line L16 (83.7222, -52.822) -> (87.9997, -52.822) projected
  line L17 (87.9997, -52.822) -> (87.9997, -52.8114) projected
  arc A5 (78.1836, -74.0042) -> (81.9836, -74.0042) centre (80.0836, -74.0042) ccw projected
  line L18 (81.9836, -74.0042) -> (81.9836, -69.6389) projected
  line L19 (81.9836, -69.6389) -> (78.1836, -69.6389) projected
  line L20 (78.1836, -69.6389) -> (78.1836, -74.0042) projected
  arc A6 (42.1836, -74.0042) -> (45.9836, -74.0042) centre (44.0836, -74.0042) ccw projected
  line L21 (45.9836, -74.0042) -> (45.9836, -69.6389) projected
  line L22 (45.9836, -69.6389) -> (42.1836, -69.6389) projected
  line L23 (42.1836, -69.6389) -> (42.1836, -74.0042) projected
  line L24 (86.061, -66.6438) -> (86.0626, -66.9863) projected
  line L25 (86.0626, -66.9863) -> (85.9765, -67.6658) projected
  line L26 (85.9765, -67.6658) -> (85.8024, -68.3282) projected
  line L27 (85.8024, -68.3282) -> (85.5433, -68.9623) projected
  line L28 (85.5433, -68.9623) -> (85.2036, -69.5571) projected
  line L29 (85.2036, -69.5571) -> (84.7893, -70.1025) projected
  line L30 (84.7893, -70.1025) -> (84.3073, -70.5891) projected
  line L31 (84.3073, -70.5891) -> (83.7659, -71.0087) projected
  line L32 (83.7659, -71.0087) -> (83.1743, -71.354) projected
  line L33 (83.1743, -71.354) -> (82.5428, -71.6191) projected
  line L34 (82.5428, -71.6191) -> (81.8821, -71.7995) projected
  line L35 (81.8821, -71.7995) -> (81.2034, -71.8922) projected
  line L36 (81.2034, -71.8922) -> (80.8609, -71.8938) projected
  line L37 (80.8609, -71.8938) -> (66.086, -71.8938) projected
  line L38 (66.086, -71.8938) -> (66.0774, -71.7633) projected
  line L39 (66.0774, -71.7633) -> (66.0098, -71.5111) projected
  line L40 (66.0098, -71.5111) -> (65.8793, -71.2851) projected
  line L41 (65.8793, -71.2851) -> (65.6947, -71.1005) projected
  line L42 (65.6947, -71.1005) -> (65.4686, -70.9699) projected
  line L43 (65.4686, -70.9699) -> (65.2165, -70.9024) projected
  line L44 (65.2165, -70.9024) -> (64.9554, -70.9024) projected
  line L45 (64.9554, -70.9024) -> (64.7033, -70.9699) projected
  line L46 (64.7033, -70.9699) -> (64.4772, -71.1005) projected
  line L47 (64.4772, -71.1005) -> (64.2926, -71.2851) projected
  line L48 (64.2926, -71.2851) -> (64.1621, -71.5111) projected
  line L49 (64.1621, -71.5111) -> (64.0945, -71.7633) projected
  line L50 (64.0945, -71.7633) -> (64.086, -71.8938) projected
  line L51 (64.086, -71.8938) -> (45.061, -71.8938) projected
  line L52 (45.061, -71.8938) -> (45.0524, -71.7633) projected
  line L53 (45.0524, -71.7633) -> (44.9848, -71.5111) projected
  line L54 (44.9848, -71.5111) -> (44.8543, -71.2851) projected
  line L55 (44.8543, -71.2851) -> (44.6697, -71.1005) projected
  line L56 (44.6697, -71.1005) -> (44.4436, -70.9699) projected
  line L57 (44.4436, -70.9699) -> (44.1915, -70.9024) projected
  line L58 (44.1915, -70.9024) -> (43.9304, -70.9024) projected
  line L59 (43.9304, -70.9024) -> (43.6783, -70.9699) projected
  line L60 (43.6783, -70.9699) -> (43.4522, -71.1005) projected
  line L61 (43.4522, -71.1005) -> (43.2676, -71.2851) projected
  line L62 (43.2676, -71.2851) -> (43.1371, -71.5111) projected
  line L63 (43.1371, -71.5111) -> (43.0695, -71.7633) projected
  line L64 (43.0695, -71.7633) -> (43.061, -71.8938) projected
  line L65 (43.061, -71.8938) -> (24.061, -71.8938) projected
  line L66 (24.061, -71.8938) -> (24.0524, -71.7633) projected
  line L67 (24.0524, -71.7633) -> (23.9848, -71.5111) projected
  line L68 (23.9848, -71.5111) -> (23.8543, -71.2851) projected
  line L69 (23.8543, -71.2851) -> (23.6697, -71.1005) projected
  line L70 (23.6697, -71.1005) -> (23.4436, -70.9699) projected
  line L71 (23.4436, -70.9699) -> (23.1915, -70.9024) projected
  line L72 (23.1915, -70.9024) -> (22.9304, -70.9024) projected
  line L73 (22.9304, -70.9024) -> (22.6783, -70.9699) projected
  line L74 (22.6783, -70.9699) -> (22.4522, -71.1005) projected
  line L75 (22.4522, -71.1005) -> (22.2676, -71.2851) projected
  line L76 (22.2676, -71.2851) -> (22.1371, -71.5111) projected
  line L77 (22.1371, -71.5111) -> (22.0695, -71.7633) projected
  line L78 (22.0695, -71.7633) -> (22.061, -71.8938) projected
  line L79 (22.061, -71.8938) -> (4.8283, -71.8187) projected
  line L80 (4.8283, -71.8187) -> (4.6526, -71.8196) projected
  line L81 (4.6526, -71.8196) -> (4.3038, -71.7753) projected
  line L82 (4.3038, -71.7753) -> (3.9638, -71.686) projected
  line L83 (3.9638, -71.686) -> (3.6384, -71.553) projected
  line L84 (3.6384, -71.553) -> (3.3331, -71.3787) projected
  line L85 (3.3331, -71.3787) -> (3.0531, -71.166) projected
  line L86 (3.0531, -71.166) -> (2.8034, -70.9186) projected
  line L87 (2.8034, -70.9186) -> (2.588, -70.6407) projected
  line L88 (2.588, -70.6407) -> (2.4108, -70.3371) projected
  line L89 (2.4108, -70.3371) -> (2.2747, -70.013) projected
  line L90 (2.2747, -70.013) -> (2.1821, -69.6738) projected
  line L91 (2.1821, -69.6738) -> (2.1346, -69.3255) projected
  line L92 (2.1346, -69.3255) -> (2.1337, -69.1497) projected
  line L93 (2.1337, -69.1497) -> (2.086, -51.9188) projected
  line L94 (2.086, -51.9188) -> (2.2165, -51.9102) projected
  line L95 (2.2165, -51.9102) -> (2.4686, -51.8427) projected
  line L96 (2.4686, -51.8427) -> (2.6947, -51.7121) projected
  line L97 (2.6947, -51.7121) -> (2.8793, -51.5276) projected
  line L98 (2.8793, -51.5276) -> (3.0098, -51.3015) projected
  line L99 (3.0098, -51.3015) -> (3.0774, -51.0493) projected
  line L100 (3.0774, -51.0493) -> (3.0774, -50.7883) projected
  line L101 (3.0774, -50.7883) -> (3.0098, -50.5361) projected
  line L102 (3.0098, -50.5361) -> (2.8793, -50.3101) projected
  line L103 (2.8793, -50.3101) -> (2.6947, -50.1255) projected
  line L104 (2.6947, -50.1255) -> (2.4686, -49.995) projected
  line L105 (2.4686, -49.995) -> (2.2165, -49.9274) projected
  line L106 (2.2165, -49.9274) -> (2.0859, -49.9188) projected
  line L107 (2.0859, -49.9188) -> (2.086, -30.8938) projected
  line L108 (2.086, -30.8938) -> (2.2165, -30.8852) projected
  line L109 (2.2165, -30.8852) -> (2.4686, -30.8177) projected
  line L110 (2.4686, -30.8177) -> (2.6947, -30.6871) projected
  line L111 (2.6947, -30.6871) -> (2.8793, -30.5026) projected
  line L112 (2.8793, -30.5026) -> (3.0098, -30.2765) projected
  line L113 (3.0098, -30.2765) -> (3.0774, -30.0243) projected
  line L114 (3.0774, -30.0243) -> (3.0774, -29.7633) projected
  line L115 (3.0774, -29.7633) -> (3.0098, -29.5111) projected
  line L116 (3.0098, -29.5111) -> (2.8793, -29.2851) projected
  line L117 (2.8793, -29.2851) -> (2.6947, -29.1005) projected
  line L118 (2.6947, -29.1005) -> (2.4686, -28.9699) projected
  line L119 (2.4686, -28.9699) -> (2.2165, -28.9024) projected
  line L120 (2.2165, -28.9024) -> (2.0859, -28.8938) projected
  line L121 (2.0859, -28.8938) -> (2.086, -9.8938) projected
  line L122 (2.086, -9.8938) -> (2.2165, -9.8852) projected
  line L123 (2.2165, -9.8852) -> (2.4687, -9.8177) projected
  line L124 (2.4687, -9.8177) -> (2.6947, -9.6871) projected
  line L125 (2.6947, -9.6871) -> (2.8793, -9.5026) projected
  line L126 (2.8793, -9.5026) -> (3.0098, -9.2765) projected
  line L127 (3.0098, -9.2765) -> (3.0774, -9.0243) projected
  line L128 (3.0774, -9.0243) -> (3.0774, -8.7633) projected
  line L129 (3.0774, -8.7633) -> (3.0098, -8.5111) projected
  line L130 (3.0098, -8.5111) -> (2.8793, -8.2851) projected
  line L131 (2.8793, -8.2851) -> (2.6947, -8.1005) projected
  line L132 (2.6947, -8.1005) -> (2.4686, -7.9699) projected
  line L133 (2.4686, -7.9699) -> (2.2165, -7.9024) projected
  line L134 (2.2165, -7.9024) -> (2.0859, -7.8938) projected
  line L135 (2.0859, -7.8938) -> (2.0859, 6.8562) projected
  line L136 (2.0859, 6.8562) -> (2.0843, 7.1986) projected
  line L137 (2.0843, 7.1986) -> (2.1705, 7.8781) projected
  line L138 (2.1705, 7.8781) -> (2.3446, 8.5406) projected
  line L139 (2.3446, 8.5406) -> (2.6037, 9.1746) projected
  line L140 (2.6037, 9.1746) -> (2.9433, 9.7694) projected
  line L141 (2.9433, 9.7694) -> (3.3576, 10.3148) projected
  line L142 (3.3576, 10.3148) -> (3.8397, 10.8015) projected
  line L143 (3.8397, 10.8015) -> (4.381, 11.221) projected
  line L144 (4.381, 11.221) -> (4.9726, 11.5663) projected
  line L145 (4.9726, 11.5663) -> (5.6041, 11.8315) projected
  line L146 (5.6041, 11.8315) -> (6.2649, 12.0119) projected
  line L147 (6.2649, 12.0119) -> (6.9435, 12.1046) projected
  line L148 (6.9435, 12.1046) -> (7.286, 12.1062) projected
  line L149 (7.286, 12.1062) -> (22.036, 12.1062) projected
  line L150 (22.036, 12.1062) -> (22.0445, 11.9757) projected
  line L151 (22.0445, 11.9757) -> (22.1121, 11.7235) projected
  line L152 (22.1121, 11.7235) -> (22.2426, 11.4974) projected
  line L153 (22.2426, 11.4974) -> (22.4272, 11.3128) projected
  line L154 (22.4272, 11.3128) -> (22.6533, 11.1823) projected
  line L155 (22.6533, 11.1823) -> (22.9054, 11.1148) projected
  line L156 (22.9054, 11.1148) -> (23.1665, 11.1148) projected
  line L157 (23.1665, 11.1148) -> (23.4186, 11.1823) projected
  line L158 (23.4186, 11.1823) -> (23.6447, 11.3128) projected
  line L159 (23.6447, 11.3128) -> (23.8293, 11.4974) projected
  line L160 (23.8293, 11.4974) -> (23.9598, 11.7235) projected
  line L161 (23.9598, 11.7235) -> (24.0274, 11.9757) projected
  line L162 (24.0274, 11.9757) -> (24.0359, 12.1062) projected
  line L163 (24.0359, 12.1062) -> (80.8109, 12.1062) projected
  line L164 (80.8109, 12.1062) -> (81.1534, 12.1078) projected
  line L165 (81.1534, 12.1078) -> (81.8329, 12.0217) projected
  line L166 (81.8329, 12.0217) -> (82.4954, 11.8476) projected
  line L167 (82.4954, 11.8476) -> (83.1294, 11.5885) projected
  line L168 (83.1294, 11.5885) -> (83.7242, 11.2489) projected
  line L169 (83.7242, 11.2489) -> (84.2696, 10.8345) projected
  line L170 (84.2696, 10.8345) -> (84.7562, 10.3525) projected
  line L171 (84.7562, 10.3525) -> (85.1758, 9.8111) projected
  line L172 (85.1758, 9.8111) -> (85.5211, 9.2196) projected
  line L173 (85.5211, 9.2196) -> (85.7862, 8.588) projected
  line L174 (85.7862, 8.588) -> (85.9667, 7.9273) projected
  line L175 (85.9667, 7.9273) -> (86.0593, 7.2486) projected
  line L176 (86.0593, 7.2486) -> (86.061, 6.9062) projected
  line L177 (86.061, 6.9062) -> (86.061, 6.8812) projected
  line L178 (86.061, 6.8812) -> (86.061, -7.8688) projected
  line L179 (86.061, -7.8688) -> (85.9305, -7.8774) projected
  line L180 (85.9305, -7.8774) -> (85.6783, -7.9449) projected
  line L181 (85.6783, -7.9449) -> (85.4522, -8.0755) projected
  line L182 (85.4522, -8.0755) -> (85.2676, -8.2601) projected
  line L183 (85.2676, -8.2601) -> (85.1371, -8.4861) projected
  line L184 (85.1371, -8.4861) -> (85.0695, -8.7383) projected
  line L185 (85.0695, -8.7383) -> (85.0695, -8.9993) projected
  line L186 (85.0695, -8.9993) -> (85.1371, -9.2515) projected
  line L187 (85.1371, -9.2515) -> (85.2676, -9.4776) projected
  line L188 (85.2676, -9.4776) -> (85.4522, -9.6621) projected
  line L189 (85.4522, -9.6621) -> (85.6783, -9.7927) projected
  line L190 (85.6783, -9.7927) -> (85.9304, -9.8602) projected
  line L191 (85.9304, -9.8602) -> (86.061, -9.8688) projected
  line L192 (86.061, -9.8688) -> (86.061, -28.8938) projected
  line L193 (86.061, -28.8938) -> (85.9305, -28.9024) projected
  line L194 (85.9305, -28.9024) -> (85.6783, -28.9699) projected
  line L195 (85.6783, -28.9699) -> (85.4522, -29.1005) projected
  line L196 (85.4522, -29.1005) -> (85.2676, -29.2851) projected
  line L197 (85.2676, -29.2851) -> (85.1371, -29.5111) projected
  line L198 (85.1371, -29.5111) -> (85.0695, -29.7633) projected
  line L199 (85.0695, -29.7633) -> (85.0695, -30.0243) projected
  line L200 (85.0695, -30.0243) -> (85.1371, -30.2765) projected
  line L201 (85.1371, -30.2765) -> (85.2676, -30.5026) projected
  line L202 (85.2676, -30.5026) -> (85.4522, -30.6871) projected
  line L203 (85.4522, -30.6871) -> (85.6783, -30.8177) projected
  line L204 (85.6783, -30.8177) -> (85.9304, -30.8852) projected
  line L205 (85.9304, -30.8852) -> (86.061, -30.8938) projected
  line L206 (86.061, -30.8938) -> (86.061, -49.8938) projected
  line L207 (86.061, -49.8938) -> (85.9305, -49.9024) projected
  line L208 (85.9305, -49.9024) -> (85.6783, -49.9699) projected
  line L209 (85.6783, -49.9699) -> (85.4522, -50.1005) projected
  line L210 (85.4522, -50.1005) -> (85.2676, -50.2851) projected
  line L211 (85.2676, -50.2851) -> (85.1371, -50.5111) projected
  line L212 (85.1371, -50.5111) -> (85.0695, -50.7633) projected
  line L213 (85.0695, -50.7633) -> (85.0695, -51.0243) projected
  line L214 (85.0695, -51.0243) -> (85.1371, -51.2765) projected
  line L215 (85.1371, -51.2765) -> (85.2676, -51.5026) projected
  line L216 (85.2676, -51.5026) -> (85.4522, -51.6872) projected
  line L217 (85.4522, -51.6872) -> (85.6783, -51.8177) projected
  line L218 (85.6783, -51.8177) -> (85.9304, -51.8853) projected
  line L219 (85.9304, -51.8853) -> (86.061, -51.8938) projected
  line L220 (86.061, -51.8938) -> (86.061, -66.6438) projected
  circle A7 centre (35.375, -47.5847) radius 1.6565 projected
  circle A8 centre (9.456, 9.6512) radius 1.2805 projected
  circle A9 centre (9.456, -36.0688) radius 1.2755 projected
  circle A10 centre (81.061, -65.3938) radius 1.2055 projected
  circle A11 centre (44.061, -29.8938) radius 1.2055 projected
  circle A12 centre (65.061, -29.8938) radius 1.2055 projected
  circle A13 centre (44.061, -50.8938) radius 1.2055 projected
  circle A14 centre (44.861, -2.7188) radius 0.8055 projected
  circle A15 centre (44.861, 4.2812) radius 0.8055 projected
  circle A16 centre (55.861, 4.2812) radius 0.8055 projected
  circle A17 centre (55.861, -2.7188) radius 0.8055 projected
  circle A18 centre (34.486, -59.2687) radius 0.6054 projected
  circle A19 centre (34.486, -62.7688) radius 0.6054 projected
  circle A20 centre (12.361, -58.5538) radius 0.5155 projected
  circle A21 centre (12.361, -61.0938) radius 0.5155 projected
  circle A22 centre (62.886, 7.8312) radius 0.5155 projected
  circle A23 centre (65.426, 7.8312) radius 0.5155 projected
  circle A24 centre (71.551, 7.8312) radius 0.5155 projected
  circle A25 centre (69.011, 7.8312) radius 0.5155 projected
  circle A26 centre (76.551, -69.6188) radius 0.5135 projected
  circle A27 centre (76.551, -67.0788) radius 0.5135 projected
  circle A28 centre (74.011, -69.6188) radius 0.5135 projected
  circle A29 centre (74.011, -67.0788) radius 0.5135 projected
  circle A30 centre (71.471, -69.6188) radius 0.5135 projected
  circle A31 centre (71.471, -67.0788) radius 0.5135 projected
  circle A32 centre (68.931, -69.6188) radius 0.5135 projected
  circle A33 centre (68.931, -67.0788) radius 0.5135 projected
  circle A34 centre (66.391, -69.6188) radius 0.5135 projected
  circle A35 centre (66.391, -67.0788) radius 0.5135 projected
  circle A36 centre (63.851, -69.6188) radius 0.5135 projected
  circle A37 centre (63.851, -67.0788) radius 0.5135 projected
  circle A38 centre (61.311, -69.6188) radius 0.5135 projected
  circle A39 centre (61.311, -67.0788) radius 0.5135 projected
  circle A40 centre (58.771, -69.6188) radius 0.5135 projected
  circle A41 centre (58.771, -67.0788) radius 0.5135 projected
  circle A42 centre (52.811, -54.4338) radius 0.5135 projected
  circle A43 centre (55.351, -54.4338) radius 0.5135 projected
  circle A44 centre (52.811, -51.8938) radius 0.5135 projected
  circle A45 centre (55.351, -51.8938) radius 0.5135 projected
  circle A46 centre (52.811, -49.3538) radius 0.5135 projected
  circle A47 centre (55.351, -49.3538) radius 0.5135 projected
  circle A48 centre (16.96, -52.0297) radius 0.5135 projected
  circle A49 centre (14.42, -52.0297) radius 0.5135 projected
  circle A50 centre (11.88, -52.0297) radius 0.5135 projected
  circle A51 centre (9.34, -52.0297) radius 0.5135 projected
  circle A52 centre (6.8, -52.0297) radius 0.5135 projected
  circle A53 centre (4.26, -52.0297) radius 0.5135 projected
  circle A54 centre (19.5, -69.8097) radius 0.5135 projected
  circle A55 centre (16.96, -69.8097) radius 0.5135 projected
  circle A56 centre (14.42, -69.8097) radius 0.5135 projected
  circle A57 centre (11.88, -69.8097) radius 0.5135 projected
  circle A58 centre (9.34, -69.8097) radius 0.5135 projected
  circle A59 centre (6.8, -69.8097) radius 0.5135 projected
  circle A60 centre (4.26, -69.8097) radius 0.5135 projected
  circle A61 centre (4.84, -3.4088) radius 0.5135 projected
  circle A62 centre (4.586, -0.8688) radius 0.5135 projected
  circle A63 centre (4.84, 1.6712) radius 0.5135 projected
  circle A64 centre (4.586, 4.2112) radius 0.5135 projected
  circle A65 centre (55.211, -68.3958) radius 0.5135 projected
  circle A66 centre (52.671, -68.6498) radius 0.5135 projected
  circle A67 centre (50.131, -68.3958) radius 0.5135 projected
  circle A68 centre (47.591, -68.6498) radius 0.5135 projected
  circle A69 centre (4.761, -12.2466) radius 0.5135 projected
  circle A70 centre (4.761, -9.351) radius 0.5135 projected
  circle A71 centre (31.811, 5.8112) radius 0.5135 projected
  circle A72 centre (32.065, 3.2712) radius 0.5135 projected
  circle A73 centre (31.811, 0.7312) radius 0.5135 projected
  circle A74 centre (32.065, -1.8088) radius 0.5135 projected
  circle A75 centre (31.811, -4.3488) radius 0.5135 projected
  circle A76 centre (32.065, -6.8888) radius 0.5135 projected
  circle A77 centre (31.811, -9.4288) radius 0.5135 projected
  circle A78 centre (32.065, -11.9688) radius 0.5135 projected
  circle A79 centre (31.811, -14.5088) radius 0.5135 projected
  circle A80 centre (32.065, -17.0488) radius 0.5135 projected
  circle A81 centre (9.351, -48.6478) radius 0.5135 projected
  circle A82 centre (6.811, -48.3938) radius 0.5135 projected
  circle A83 centre (4.271, -48.6478) radius 0.5135 projected
  circle A84 centre (41.136, -59.441) radius 0.5135 projected
  circle A85 centre (41.136, -62.3366) radius 0.5135 projected
  circle A86 centre (36.899, -59.6497) radius 0.5055 projected
  circle A87 centre (36.899, -62.1897) radius 0.5055 projected
  circle A88 centre (21.8126, -20.375) radius 0.5055 projected
  circle A89 centre (24.3526, -20.375) radius 0.5055 projected
  circle A90 centre (21.8126, -17.835) radius 0.5055 projected
  circle A91 centre (24.3526, -17.835) radius 0.5055 projected
  circle A92 centre (21.8126, -15.295) radius 0.5055 projected
  circle A93 centre (24.3526, -15.295) radius 0.5055 projected
  circle A94 centre (21.8126, -12.755) radius 0.5055 projected
  circle A95 centre (24.3526, -12.755) radius 0.5055 projected
  circle A96 centre (21.8126, -10.215) radius 0.5055 projected
  circle A97 centre (24.3526, -10.215) radius 0.5055 projected
  circle A98 centre (21.8126, -7.675) radius 0.5055 projected
  circle A99 centre (24.3526, -7.675) radius 0.5055 projected
  circle A100 centre (21.8126, -5.135) radius 0.5055 projected
  circle A101 centre (24.3526, -5.135) radius 0.5055 projected
  circle A102 centre (21.8126, -2.595) radius 0.5055 projected
  circle A103 centre (24.3526, -2.595) radius 0.5055 projected
  circle A104 centre (21.8126, -0.055) radius 0.5055 projected
  circle A105 centre (24.3526, -0.055) radius 0.5055 projected
  circle A106 centre (21.8126, 2.485) radius 0.5055 projected
  circle A107 centre (24.3526, 2.485) radius 0.5055 projected
  circle A108 centre (24.3506, -39.495) radius 0.5055 projected
  circle A109 centre (21.8106, -39.495) radius 0.5055 projected
  circle A110 centre (24.3506, -42.035) radius 0.5055 projected
  circle A111 centre (21.8106, -42.035) radius 0.5055 projected
  circle A112 centre (24.3506, -44.575) radius 0.5055 projected
  circle A113 centre (21.8106, -44.575) radius 0.5055 projected
  circle A114 centre (24.3506, -47.115) radius 0.5055 projected
  circle A115 centre (21.8106, -47.115) radius 0.5055 projected
  circle A116 centre (24.3506, -49.655) radius 0.5055 projected
  circle A117 centre (21.8106, -49.655) radius 0.5055 projected
  circle A118 centre (24.3506, -52.195) radius 0.5055 projected
  circle A119 centre (21.8106, -52.195) radius 0.5055 projected
  circle A120 centre (24.3506, -54.735) radius 0.5055 projected
  circle A121 centre (21.8106, -54.735) radius 0.5055 projected
  circle A122 centre (24.3506, -57.275) radius 0.5055 projected
  circle A123 centre (21.8106, -57.275) radius 0.5055 projected
  circle A124 centre (24.3506, -59.815) radius 0.5055 projected
  circle A125 centre (21.8106, -59.815) radius 0.5055 projected
  circle A126 centre (24.3506, -62.355) radius 0.5055 projected
  circle A127 centre (21.8106, -62.355) radius 0.5055 projected
  circle A128 centre (63.8376, -62.355) radius 0.5055 projected
  circle A129 centre (66.3776, -62.355) radius 0.5055 projected
  circle A130 centre (63.8376, -59.815) radius 0.5055 projected
  circle A131 centre (66.3776, -59.815) radius 0.5055 projected
  circle A132 centre (63.8376, -57.275) radius 0.5055 projected
  circle A133 centre (66.3776, -57.275) radius 0.5055 projected
  circle A134 centre (63.8376, -54.735) radius 0.5055 projected
  circle A135 centre (66.3776, -54.735) radius 0.5055 projected
  circle A136 centre (63.8376, -52.195) radius 0.5055 projected
  circle A137 centre (66.3776, -52.195) radius 0.5055 projected
  circle A138 centre (63.8376, -49.655) radius 0.5055 projected
  circle A139 centre (66.3776, -49.655) radius 0.5055 projected
  circle A140 centre (63.8376, -47.115) radius 0.5055 projected
  circle A141 centre (66.3776, -47.115) radius 0.5055 projected
  circle A142 centre (63.8376, -44.575) radius 0.5055 projected
  circle A143 centre (66.3776, -44.575) radius 0.5055 projected
  circle A144 centre (63.8376, -42.035) radius 0.5055 projected
  circle A145 centre (66.3776, -42.035) radius 0.5055 projected
  circle A146 centre (63.8376, -39.495) radius 0.5055 projected
  circle A147 centre (66.3776, -39.495) radius 0.5055 projected
  circle A148 centre (66.3776, 2.485) radius 0.5055 projected
  circle A149 centre (63.8376, 2.485) radius 0.5055 projected
  circle A150 centre (66.3776, -0.055) radius 0.5055 projected
  circle A151 centre (63.8376, -0.055) radius 0.5055 projected
  circle A152 centre (66.3776, -2.595) radius 0.5055 projected
  circle A153 centre (63.8376, -2.595) radius 0.5055 projected
  circle A154 centre (66.3776, -5.135) radius 0.5055 projected
  circle A155 centre (63.8376, -5.135) radius 0.5055 projected
  circle A156 centre (66.3776, -7.675) radius 0.5055 projected
  circle A157 centre (63.8376, -7.675) radius 0.5055 projected
  circle A158 centre (66.3776, -10.215) radius 0.5055 projected
  circle A159 centre (63.8376, -10.215) radius 0.5055 projected
  circle A160 centre (66.3776, -12.755) radius 0.5055 projected
  circle A161 centre (63.8376, -12.755) radius 0.5055 projected
  circle A162 centre (66.3776, -15.295) radius 0.5055 projected
  circle A163 centre (63.8376, -15.295) radius 0.5055 projected
  circle A164 centre (66.3776, -17.835) radius 0.5055 projected
  circle A165 centre (63.8376, -17.835) radius 0.5055 projected
  circle A166 centre (66.3776, -20.375) radius 0.5055 projected
  circle A167 centre (63.8376, -20.375) radius 0.5055 projected
  circle A168 centre (28.506, -1.7788) radius 0.5055 projected
  circle A169 centre (28.506, 5.8412) radius 0.5055 projected
  circle A170 centre (28.506, 3.3012) radius 0.5055 projected
  circle A171 centre (28.506, 0.7612) radius 0.5055 projected
  circle A172 centre (28.506, -4.3188) radius 0.5055 projected
  circle A173 centre (28.506, -6.8588) radius 0.5055 projected
  circle A174 centre (28.506, -9.3988) radius 0.5055 projected
  circle A175 centre (28.506, -11.9388) radius 0.5055 projected
  circle A176 centre (28.506, -14.4788) radius 0.5055 projected
  circle A177 centre (28.506, -17.0188) radius 0.5055 projected
  circle A178 centre (28.506, -19.5588) radius 0.5055 projected
  circle A179 centre (28.506, -22.0988) radius 0.5055 projected
  circle A180 centre (28.506, -24.6388) radius 0.5055 projected
  circle A181 centre (28.506, -27.1788) radius 0.5055 projected
  circle A182 centre (28.506, -29.7188) radius 0.5055 projected
  circle A183 centre (28.506, -32.2588) radius 0.5055 projected
  circle A184 centre (8.186, -32.2588) radius 0.5055 projected
  circle A185 centre (8.186, -29.7188) radius 0.5055 projected
  circle A186 centre (8.186, -27.1788) radius 0.5055 projected
  circle A187 centre (8.186, -24.6388) radius 0.5055 projected
  circle A188 centre (8.186, -22.0988) radius 0.5055 projected
  circle A189 centre (8.186, -19.5588) radius 0.5055 projected
  circle A190 centre (8.186, -17.0188) radius 0.5055 projected
  circle A191 centre (8.186, -14.4788) radius 0.5055 projected
  circle A192 centre (8.186, -11.9388) radius 0.5055 projected
  circle A193 centre (8.186, -9.3988) radius 0.5055 projected
  circle A194 centre (8.186, -6.8588) radius 0.5055 projected
  circle A195 centre (8.186, -4.3188) radius 0.5055 projected
  circle A196 centre (9.021, -43.8938) radius 0.5055 projected
  circle A197 centre (11.561, -43.8938) radius 0.5055 projected
  circle A198 centre (14.101, -43.8938) radius 0.5055 projected
  circle A199 centre (35.381, -7.1738) radius 0.4555 projected
  circle A200 centre (37.921, -9.7138) radius 0.4555 projected
  circle A201 centre (37.921, -7.1738) radius 0.4555 projected
  circle A202 centre (78.561, -42.7338) radius 0.4555 projected
  circle A203 centre (81.101, -42.7338) radius 0.4555 projected
  circle A204 centre (78.561, -40.1938) radius 0.4555 projected
  circle A205 centre (81.101, -40.1938) radius 0.4555 projected
  circle A206 centre (78.561, -37.6538) radius 0.4555 projected
  circle A207 centre (81.101, -37.6538) radius 0.4555 projected
  circle A208 centre (78.561, -35.1138) radius 0.4555 projected
  circle A209 centre (81.101, -35.1138) radius 0.4555 projected
  circle A210 centre (37.921, -42.7338) radius 0.4555 projected
  circle A211 centre (37.921, -37.6538) radius 0.4555 projected
  circle A212 centre (37.921, -40.1938) radius 0.4555 projected
  circle A213 centre (35.381, -40.1938) radius 0.4555 projected
  circle A214 centre (35.381, -42.7338) radius 0.4555 projected
  circle A215 centre (37.921, 10.6062) radius 0.4555 projected
  circle A216 centre (35.381, 8.0662) radius 0.4555 projected
  circle A217 centre (35.381, 10.6062) radius 0.4555 projected
  circle A218 centre (37.921, 8.0662) radius 0.4555 projected
  circle A219 centre (37.921, 5.5262) radius 0.4555 projected
  circle A220 centre (35.381, 5.5262) radius 0.4555 projected
  circle A221 centre (37.921, 2.9862) radius 0.4555 projected
  circle A222 centre (35.381, 2.9862) radius 0.4555 projected
  circle A223 centre (37.921, 0.4462) radius 0.4555 projected
  circle A224 centre (35.381, 0.4462) radius 0.4555 projected
  circle A225 centre (37.921, -2.0938) radius 0.4555 projected
  circle A226 centre (35.381, -2.0938) radius 0.4555 projected
  circle A227 centre (35.381, -4.6338) radius 0.4555 projected
  circle A228 centre (37.921, -4.6338) radius 0.4555 projected
  circle A229 centre (35.381, -9.7138) radius 0.4555 projected
  circle A230 centre (37.921, -12.2538) radius 0.4555 projected
  circle A231 centre (35.381, -12.2538) radius 0.4555 projected
  circle A232 centre (37.921, -14.7938) radius 0.4555 projected